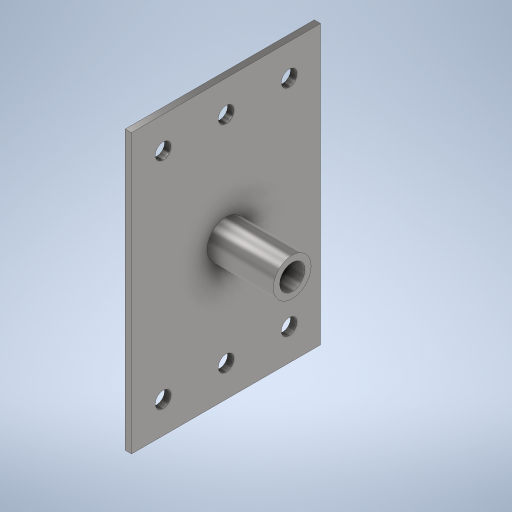
# Autodesk Inventor part: ax4_holder
Saved by Autodesk Inventor 2024 (Build 280153000, 153)
## iProperties
Created: 2025-12-19
Part Number: ax4_holder
Material: Iron, Malleable
Document SubType Name: Modeling
Designer: schar
Density: 7.15 g/cm^3
Appearance: Semi-Polished
Author: schar
Autodesk Inventor part; units mm, degrees
ref_plane "YZ Plane" through (0, 0, 0) normal (1, 0, 0) x (0, 1, 0)
ref_plane "XZ Plane" through (0, 0, 0) normal (0, 1, 0) x (-1, 0, 0)
ref_plane "XY Plane" through (0, 0, 0) normal (0, 0, 1) x (1, 0, 0)
sketch "Sketch1" plane through (0, 0, 0) normal (1, 0, 0) x (0, 1, 0)
  line L0 (44.15, 30) -> (-44.15, 30)
  line L1 (-44.15, 30) -> (-44.15, -30)
  line L2 (-44.15, -30) -> (44.15, -30)
  line L3 (44.15, -30) -> (44.15, 30)
  line L4 (44.15, 30) -> (-44.15, -30) construction
  line L5 (-44.15, 30) -> (44.15, -30) construction
  circle A0 centre (0, 0) radius 4
  circle A1 centre (0, 0) radius 6
  line L6 (44.15, 30) -> (44.15, 20)
  line L7 (44.15, 20) -> (34.15, 20)
  line L8 (44.15, -30) -> (44.15, -20)
  line L9 (44.15, -20) -> (34.15, -20)
  line L10 (-44.15, 30) -> (-44.15, 20)
  line L11 (-44.15, 20) -> (-34.15, 20)
  line L12 (-44.15, -30) -> (-44.15, -20)
  line L13 (-44.15, -20) -> (-34.15, -20)
  line L14 (-44.15, 0) -> (-34.15, 0)
  line L15 (44.15, 0) -> (34.15, 0)
  circle A2 centre (34.15, 20) radius 2.5
  circle A3 centre (34.15, 0) radius 2.5
  circle A4 centre (34.15, -20) radius 2.5
  circle A5 centre (-34.15, 20) radius 2.5
  circle A6 centre (-34.15, 0) radius 2.5
  circle A7 centre (-34.15, -20) radius 2.5
  dimension "d0" = 88.3
  dimension "d1" = 60
  dimension "d2" = 8
  dimension "d3" = 12
  dimension "d4" = 10
  dimension "d5" = 10
  dimension "d6" = 10
  dimension "d7" = 10
  dimension "d8" = 10
  dimension "d9" = 10
  dimension "d10" = 10
  dimension "d11" = 10
  dimension "d12" = 10
  dimension "d13" = 10
  dimension "d14" = 5
  dimension "d15" = 5
  dimension "d16" = 5
  dimension "d17" = 5
  dimension "d18" = 5
  dimension "d19" = 5
  constraints: 32 end point, 8 centre point, 8 coincident, 5 perpendicular, 4 midpoint, 4 point on line, 3 horizontal, 2 parallel
  measures "d0" distance of L2.end L1.end
  measures "d1" distance of L1.end L0.end
  measures "d2" diameter of A0
  measures "d3" diameter of A1
  measures "d4" distance of L0.start L6.end
  measures "d5" distance of L6.end L7.end
  measures "d6" distance of L2.end L8.end
  measures "d7" distance of L8.end L9.end
  measures "d8" distance of L0.end L10.end
  measures "d9" distance of L10.end L11.end
  measures "d10" distance of L1.end L12.end
  measures "d11" distance of L12.end L13.end
  measures "d12" distance of L14.start L14.end
  measures "d13" distance of L15.start L15.end
  measures "d14" diameter of A2
  measures "d15" diameter of A3
  measures "d16" diameter of A4
  measures "d17" diameter of A5
  measures "d18" diameter of A6
  measures "d19" diameter of A7
extrude "Extrusion1" add sketch "Sketch1" along normal blind 2 contours L3 L2 L1 L0
sketch "Sketch2" plane through (2, 0, 0) normal (1, 0, 0) x (0, 0, -1)
  circle A0 centre (0, 0) radius 6
  circle A1 centre (0, 0) radius 4
  dimension "d22" = 12
  dimension "d23" = 8
  constraints: 2 centre point, 2 coincident
  measures "d22" diameter of A0
  measures "d23" diameter of A1
extrude "Extrusion2" add sketch "Sketch2" along normal blind 21 and the other way blind 2
ref_plane "Work Plane1" through (2, 0, -6) normal (0, 0, -1) x (-1, 0, 0)
sketch "Sketch3" plane through (2, 0, -6) normal (0, 0, -1) x (-1, 0, 0)
  line L0 (-21, 6) -> (-21, -6) projected
  line L1 (-21, 0) -> (-10, 0)
  circle A0 centre (-10, 0) radius 2
  point P0 (2, 0)
  dimension "d28" = 11
  dimension "d29" = 4
  constraints: 2 end point, 1 centre point, 1 coincident, 1 horizontal, 1 midpoint
  measures "d28" distance of L1.start L1.end
  measures "d29" diameter of A0
extrude "Extrusion3" cut sketch "Sketch3" against normal blind 5
thread "Thread1" size "M4x0.7" class "6H" standard "ANSI Metric M Profile" length 15
body "Solid1"
